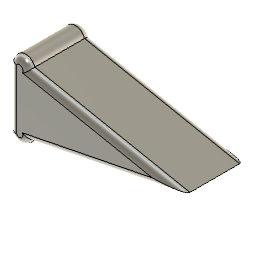
wedgeOfPower (Autodesk Fusion 360 design; units mm, degrees)
Autodesk Fusion 360 part; units mm, degrees
sketch "Sketch1" plane through (0, 0, 0) normal (0, 1, 0) x (1, 0, 0)
  line L0 (25, 0) -> (0, -5)
  line L1 (25, 0) -> (0, 5)
  arc A0 (-3, -5) -> (0, -5) centre (-1.5, -4.5) ccw
  arc A1 (0, 5) -> (-3, 5) centre (-1.5, 4.5) ccw
  line L2 (-3, -5) -> (-3, 5)
  dimension "d1" = 3
  constraint vertical L2
  measures "d1" distance of L1.end A1.end
extrude "Extrude1" add sketch "Sketch1" along normal blind 10
fillet "Fillet1" radius 1 5 edges at (12.5, 10, 2.5) (12.5, 10, -2.5) (-1.5, 10, 6.0811) (-3, 10, 0) (-1.5, 10, -6.0811)
fillet "Fillet2" radius 1 5 edges at (12.5, 0, 2.5) (-1.5, 0, 6.0811) (-3, 0, 0) (-1.5, 0, -6.0811) (12.5, 0, -2.5)
